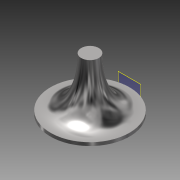
# Autodesk Inventor part: Impeller
Saved by Autodesk Inventor 2018.2 (Build 222227000, 227)
## iProperties
Created: 2018-02-01
Part Number: Impeller
Material: Steel, Galvanized
Document SubType Name: Modeling
Designer: Rus
Density: 7.85 g/cm^3
Appearance: Semi-Polished
Author: Rus
Autodesk Inventor part; units mm, degrees
ref_plane "YZ Plane" through (0, 0, 0) normal (1, 0, 0) x (0, 1, 0)
ref_plane "XZ Plane" through (0, 0, 0) normal (0, 1, 0) x (-1, 0, 0)
ref_plane "XY Plane" through (0, 0, 0) normal (0, 0, 1) x (1, 0, 0)
sketch "Sketch1" plane through (0, 0, 0) normal (0, 1, 0) x (-1, 0, 0)
  circle A0 centre (0, 0) radius 38.1
  line L0 (0, 0) -> (0, -38.1) construction
  dimension "d0" = 76.2
  constraints: 2 end point, 1 coincident, 1 vertical, 1 vertical alignment, 2 other
ref_plane "Work Plane1" through (0, 0, 0) normal (0, 0, -1) x (-1, 0, 0)
ref_plane "Work Plane2" through (0, 0, -38.1) normal (0, 0, -1) x (-1, 0, 0)
extrude "Extrusion1" add sketch "Sketch1" along normal blind 3.175
sketch "Sketch2" plane through (0, 0, 0) normal (0, 0, -1) x (-1, 0, 0)
  line L0 (38.1, 3.175) -> (-38.1, 3.175) projected
  line L1 (0, 3.175) -> (0, 50.8)
  line L2 (0, 50.8) -> (-8.4667, 50.8)
  line L3 (-38.1, 0) -> (38.1, 0) projected
  line L4 (-38.1, 3.175) -> (-29.6333, 3.175) construction
  line L5 (-29.6333, 3.175) -> (-27.7702, 5.0382) construction
  line L6 (-27.7702, 5.0382) -> (-8.4667, 7.4083) construction
  line L7 (-8.4667, 7.4083) -> (-8.4667, 50.8) construction
  spline S0 degree 4 poles (-38.1, 3.175) (-29.6333, 3.175) (-27.7702, 5.0382) (-8.4667, 7.4083) (-8.4667, 50.8) knots 0 0 0 0 0 1 1 1 1 1
  point P0 (0, 0)
  dimension "d5" = 8.4667
  dimension "d13" = 50.8
  dimension "d17" = 8.4667
  dimension "d18" = 45
  dimension "d19" = 7
  dimension "d20" = 4.2333
  constraints: 4 end point, 2 horizontal, 1 midpoint, 1 point on line, 1 vertical, 3 other
  measures "d5" distance of L1.end L2.end
  measures "d13" distance from line of L1.end L3
  measures "d17" horizontal distance of L3.start L4.end
  measures "d18" angle of L0 L5
  measures "d19" angle of L0 L6
  measures "d20" distance from line of L0 L6.end
revolve "Revolution1" add sketch "Sketch2" angle 360 about axis through (0, 3.175, 0) along (0, 1, 0)
body "Solid1"
